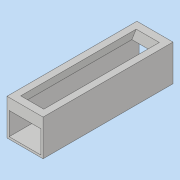
# Autodesk Inventor part: MidshipsUnibody
Saved by Autodesk Inventor 2017.3 (Build 213256000, 256)
## iProperties
Created: 2018-07-15
Part Number: MidshipsUnibody
Material: Generic
Document SubType Name: Modeling
Designer: Derek Wider
Density: 1 g/cm^3
Appearance: Default
Author: Derek Wider
Autodesk Inventor part; units mm, degrees
ref_plane "YZ Plane" through (0, 0, 0) normal (1, 0, 0) x (0, 1, 0)
ref_plane "XZ Plane" through (0, 0, 0) normal (0, 1, 0) x (-1, 0, 0)
ref_plane "XY Plane" through (0, 0, 0) normal (0, 0, 1) x (1, 0, 0)
sketch "Sketch1" plane through (0, 0, 0) normal (0, 1, 0) x (-1, 0, 0)
  line L0 (0, 0) -> (31.75, 0)
  line L1 (31.75, 0) -> (31.75, -114.3)
  line L2 (31.75, -114.3) -> (0, -114.3)
  line L3 (0, -114.3) -> (0, 0)
  dimension "d0" = 31.75
  dimension "d1" = 114.3
  constraints: 8 end point, 2 parallel, 1 horizontal, 1 perpendicular
  measures "d0" distance of L0.start L0.end
  measures "d1" distance of L2.end L0.start
extrude "Extrusion1" add sketch "Sketch1" along normal blind 31.75
shell "Shell1" thickness 1.905 removed faces 3 at (-10.5833, 10.5833, 0) at (-21.1667, 21.1667, -114.3) at (-10.5833, 31.75, -38.1)
sketch "Sketch2" plane through (-31.75, 0, 0) normal (0, 0, 1) x (1, 0, 0)
  line L0 (1.905, 1.905) -> (1.905, 31.75) projected
  line L1 (29.845, 31.75) -> (29.845, 1.905) projected
  line L2 (1.905, 31.75) -> (5.715, 31.75)
  line L3 (5.715, 31.75) -> (1.905, 21.8784)
  line L4 (1.905, 31.75) -> (1.905, 1.905) projected
  line L5 (29.845, 31.75) -> (26.035, 31.75)
  line L6 (26.035, 31.75) -> (29.845, 21.8784)
  point P0 (31.75, 0)
  dimension "d5" = 3.81
  constraints: 8 end point, 3 point on line, 2 equal length, 1 horizontal
  measures "d5" distance of L1.start L5.end
extrude "Extrusion2" add sketch "Sketch2" against normal up to surface (114.3 mm away)
sketch "Sketch4" plane through (-31.75, 0, 0) normal (0, 0, 1) x (1, 0, 0)
  line L0 (1.905, 21.8784) -> (5.715, 31.75) projected
  line L1 (29.845, 21.8784) -> (26.035, 31.75) projected
  line L2 (5.715, 31.75) -> (26.035, 31.75)
  line L3 (1.905, 21.8784) -> (29.845, 21.8784)
  point P0 (31.75, 0)
  constraints: 4 end point, 2 horizontal, 1 point on line
extrude "Extrusion3" add sketch "Sketch4" against normal blind 6.35
sketch "Sketch5" plane through (0, 0, -114.3) normal (0, 0, -1) x (-1, 0, 0)
  line L0 (26.035, 31.75) -> (29.845, 21.8784) projected
  line L1 (26.035, 31.75) -> (5.715, 31.75) projected
  line L2 (1.905, 21.8784) -> (5.715, 31.75) projected
  line L3 (1.905, 21.8784) -> (29.845, 21.8784) projected
  point P0 (0, 0)
extrude "Extrusion4" add sketch "Sketch5" against normal blind 6.35
body "Solid1"
